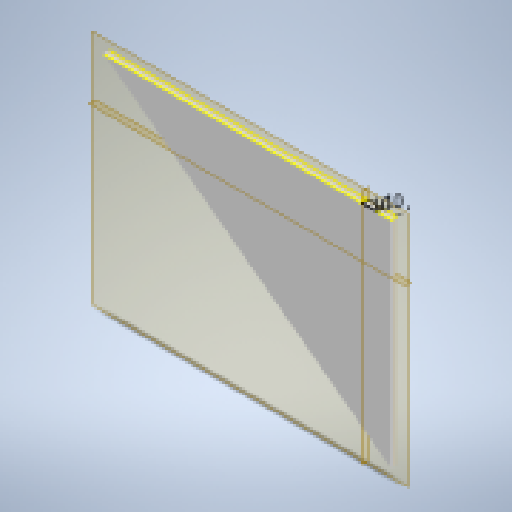
# Autodesk Inventor part: Ребро жёсткости для крепления хвоста
Saved by Autodesk Inventor 2023.2 (Build 272271030, 271C)
## iProperties
Created: 2024-03-15
Part Number: Ребро жёсткости для крепления хвоста
Material: Типовые
Document SubType Name: Modeling
Designer: I9232
Density: 1 g/cm^3
Appearance: По умолчанию
Author: I9232
Autodesk Inventor part; units mm, degrees
sketch "Эскиз1" plane through (0, 0, 0) normal (0, 0, 1) x (1, 0, 0)
  line L0 (-180, 35) -> (20, 35)
  line L1 (20, 35) -> (20, -115)
  line L2 (20, -115) -> (-180, 35)
  dimension "d4" = 150
  dimension "d5" = 200
  constraints: 6 end point, 1 perpendicular
  measures "d4" distance of L0.end L1.end
  measures "d5" distance of L0.start L0.end
extrude "Выдавливание1" add sketch "Эскиз1" along normal mid plane 4
sketch "Эскиз2" plane through (-180, 35, 2) normal (0, 1, 0) x (1, 0, 0)
  line L0 (200, 0) -> (0, 0) projected
  line L1 (0, 4) -> (200, 4) projected
  line L2 (190, 0) -> (180, 0)
  line L3 (180, 0) -> (180, 4)
  line L4 (180, 4) -> (190, 4)
  line L5 (190, 4) -> (190, 0)
  line L6 (200, 4) -> (200, 0) projected
  line L7 (170, 0) -> (160, 0)
  line L8 (160, 0) -> (160, 4)
  line L9 (160, 4) -> (170, 4)
  line L10 (170, 4) -> (170, 0)
  line L11 (-310, 0) -> (-320, 0)
  line L12 (-320, 0) -> (-320, 4)
  line L13 (-320, 4) -> (-310, 4)
  line L14 (-310, 4) -> (-310, 0)
  line L15 (-330, 0) -> (-340, 0)
  line L16 (-340, 0) -> (-340, 4)
  line L17 (-340, 4) -> (-330, 4)
  line L18 (-330, 4) -> (-330, 0)
  line L19 (110, 0) -> (110, 4)
  line L20 (120, 0) -> (110, 0)
  line L21 (110, 4) -> (120, 4)
  line L22 (120, 4) -> (120, 0)
  line L23 (130, 0) -> (130, 4)
  line L24 (130, 4) -> (140, 4)
  line L25 (140, 4) -> (140, 0)
  line L26 (140, 0) -> (130, 0)
  line L27 (60, 0) -> (60, 4)
  line L28 (70, 0) -> (60, 0)
  line L29 (60, 4) -> (70, 4)
  line L30 (70, 4) -> (70, 0)
  line L31 (80, 0) -> (80, 4)
  line L32 (80, 4) -> (90, 4)
  line L33 (90, 4) -> (90, 0)
  line L34 (90, 0) -> (80, 0)
  line L35 (10, 0) -> (10, 4)
  line L36 (20, 0) -> (10, 0)
  line L37 (10, 4) -> (20, 4)
  line L38 (20, 4) -> (20, 0)
  line L39 (30, 0) -> (30, 4)
  line L40 (30, 4) -> (40, 4)
  line L41 (40, 4) -> (40, 0)
  line L42 (40, 0) -> (30, 0)
  point P0 (180, 2)
  point P1 (180, 2)
  point P2 (170, 2)
  point P3 (-320, 2)
  point P4 (-330, 2)
  point P5 (120, 2)
  point P6 (130, 2)
  point P7 (70, 2)
  point P8 (80, 2)
  point P9 (20, 2)
  point P10 (30, 2)
  dimension "d6" = 10
  dimension "d7" = 10
  dimension "d8" = 10
  dimension "d9" = 10
  dimension "d12" = 500
  dimension "d19" = 50
  constraints: 80 end point, 4 horizontal, 4 parallel, 4 point on line, 2 midpoint, 2 perpendicular, 72 other
  measures "d6" distance of L4.end L3.end
  measures "d7" distance between parallel lines of L5 L6
  measures "d8" distance of L9.end L8.end
  measures "d9" distance of point (180, 2) point (170, 2)
  measures "d12" distance of L2.start L11.start
  measures "d19" distance of L2.start L25.end
extrude "Выдавливание2" add sketch "Эскиз2" along normal blind 3 contours L0 L3 L1 L5 | L0 L8 L1 L10 | L0 L23 L1 L25 | L0 L19 L1 L22 | L0 L31 L1 L33 | L0 L27 L1 L30 | L0 L39 L1 L41 | L0 L35 L1 L38
sketch "Эскиз3" plane through (20, -115, 2) normal (1, 0, 0) x (0, 0, -1)
  line L0 (0, 0) -> (0, 150) projected
  line L1 (4, 0) -> (4, 150) projected
  line L2 (0, 11.5) -> (4, 11.5)
  line L3 (4, 11.5) -> (4, 21.5)
  line L4 (4, 21.5) -> (0, 21.5)
  line L5 (0, 21.5) -> (0, 11.5)
  line L6 (0, 0) -> (4, 0) projected
  line L7 (0, 31.5) -> (4, 31.5)
  line L8 (4, 31.5) -> (4, 41.5)
  line L9 (4, 41.5) -> (0, 41.5)
  line L10 (0, 41.5) -> (0, 31.5)
  line L11 (0, 61.5) -> (4, 61.5)
  line L12 (4, 61.5) -> (4, 71.5)
  line L13 (4, 71.5) -> (0, 71.5)
  line L14 (0, 71.5) -> (0, 61.5)
  line L15 (0, 81.5) -> (4, 81.5)
  line L16 (4, 81.5) -> (4, 91.5)
  line L17 (4, 91.5) -> (0, 91.5)
  line L18 (0, 91.5) -> (0, 81.5)
  line L19 (0, 111.5) -> (4, 111.5)
  line L20 (4, 111.5) -> (4, 121.5)
  line L21 (4, 121.5) -> (0, 121.5)
  line L22 (0, 121.5) -> (0, 111.5)
  line L23 (0, 131.5) -> (4, 131.5)
  line L24 (4, 131.5) -> (4, 141.5)
  line L25 (4, 141.5) -> (0, 141.5)
  line L26 (0, 141.5) -> (0, 131.5)
  point P0 (2, 115)
  point P1 (0, 141.5)
  point P2 (0, 91.5)
  point P3 (0, 121.5)
  point P4 (0, 71.5)
  point P5 (0, 61.5)
  point P6 (4, 61.5)
  point P7 (0, 41.5)
  point P8 (4, 31.5)
  point P9 (0, 21.5)
  point P10 (4, 11.5)
  dimension "d26" = 11.5
  dimension "d27" = 10
  dimension "d28" = 10
  dimension "d29" = 10
  dimension "d32" = 50
  constraints: 48 end point, 4 parallel, 4 point on line, 2 horizontal, 2 perpendicular, 1 vertical, 32 other
  measures "d26" distance between parallel lines of L2 L6
  measures "d27" distance of L3.end L2.end
  measures "d28" distance of L9.end L7.start
  measures "d29" distance between parallel lines of L7 L4
  measures "d32" distance of L2.start L11.start
extrude "Выдавливание3" add sketch "Эскиз3" along normal blind 4 contours L0 L4 L1 L2 | L0 L9 L1 L7 | L0 L13 L1 L11 | L0 L17 L1 L15 | L0 L21 L1 L19 | L0 L25 L1 L23
sketch "Эскиз4" plane through (0, 0, 2) normal (0, 0, 1) x (1, 0, 0)
  line L0 (5.1, -89.95) -> (5.1, -87.05)
  line L1 (20, -87.05) -> (20, -89.95)
  line L2 (20, -93.5) -> (20, -83.5) projected
  line L3 (5.1, -88.5) -> (20, -88.5) construction
  line L4 (20, -83.5) -> (20, -93.5) projected
  line L5 (10.1, -91.3) -> (11.9, -91.3)
  line L6 (11.9, -85.7) -> (10.1, -85.7)
  line L7 (20, -89.95) -> (11.9, -89.95)
  line L8 (10.1, -89.95) -> (5.1, -89.95)
  line L9 (10.1, -85.7) -> (10.1, -87.05)
  line L10 (10.1, -89.95) -> (10.1, -91.3)
  line L11 (11.9, -91.3) -> (11.9, -89.95)
  line L12 (11.9, -87.05) -> (11.9, -85.7)
  line L13 (5.1, -87.05) -> (10.1, -87.05)
  line L14 (11.9, -87.05) -> (20, -87.05)
  line L15 (10.1, -39.95) -> (10.1, -41.3)
  line L16 (10.1, -35.7) -> (10.1, -37.05)
  line L17 (10.1, -41.3) -> (11.9, -41.3)
  line L18 (11.9, -41.3) -> (11.9, -39.95)
  line L19 (11.9, -35.7) -> (10.1, -35.7)
  line L20 (11.9, -37.05) -> (11.9, -35.7)
  line L21 (5.1, -38.5) -> (20, -38.5) construction
  line L22 (20, -39.95) -> (11.9, -39.95)
  line L23 (11.9, -37.05) -> (20, -37.05)
  line L24 (20, -37.05) -> (20, -39.95)
  line L25 (5.1, -37.05) -> (10.1, -37.05)
  line L26 (5.1, -39.95) -> (5.1, -37.05)
  line L27 (10.1, -39.95) -> (5.1, -39.95)
  line L28 (10.1, 10.05) -> (10.1, 8.7)
  line L29 (10.1, 14.3) -> (10.1, 12.95)
  line L30 (10.1, 8.7) -> (11.9, 8.7)
  line L31 (11.9, 8.7) -> (11.9, 10.05)
  line L32 (11.9, 14.3) -> (10.1, 14.3)
  line L33 (11.9, 12.95) -> (11.9, 14.3)
  line L34 (5.1, 11.5) -> (20, 11.5) construction
  line L35 (20, 10.05) -> (11.9, 10.05)
  line L36 (11.9, 12.95) -> (20, 12.95)
  line L37 (20, 12.95) -> (20, 10.05)
  line L38 (5.1, 12.95) -> (10.1, 12.95)
  line L39 (5.1, 10.05) -> (5.1, 12.95)
  line L40 (10.1, 10.05) -> (5.1, 10.05)
  line L41 (-6.454, 35) -> (-3.546, 35)
  line L42 (-3.546, 20.1) -> (-6.446, 20.1)
  line L43 (-4.996, 20.1) -> (-5, 35) construction
  line L44 (0, 35) -> (-10, 35) projected
  line L45 (-2.196, 25.1) -> (-2.196, 26.9)
  line L46 (-7.796, 26.9) -> (-7.796, 25.1)
  line L47 (-6.446, 20.1) -> (-6.446, 25.1)
  line L48 (-6.454, 26.9) -> (-6.454, 35)
  line L49 (-7.796, 25.1) -> (-6.446, 25.1)
  line L50 (-3.546, 25.1) -> (-2.196, 25.1)
  line L51 (-2.196, 26.9) -> (-3.546, 26.9)
  line L52 (-6.454, 26.9) -> (-7.796, 26.9)
  line L53 (-3.546, 35) -> (-3.546, 26.9)
  line L54 (-3.546, 25.1) -> (-3.546, 20.1)
  line L55 (-53.546, 25.1) -> (-52.196, 25.1)
  line L56 (-57.796, 26.9) -> (-57.796, 25.1)
  line L57 (-56.454, 26.9) -> (-57.796, 26.9)
  line L58 (-52.196, 25.1) -> (-52.196, 26.9)
  line L59 (-52.196, 26.9) -> (-53.546, 26.9)
  line L60 (-54.996, 20.1) -> (-55, 35) construction
  line L61 (-53.546, 35) -> (-53.546, 26.9)
  line L62 (-56.454, 26.9) -> (-56.454, 35)
  line L63 (-56.454, 35) -> (-53.546, 35)
  line L64 (-53.546, 20.1) -> (-56.446, 20.1)
  line L65 (-53.546, 25.1) -> (-53.546, 20.1)
  line L66 (-56.446, 20.1) -> (-56.446, 25.1)
  line L67 (-57.796, 25.1) -> (-56.446, 25.1)
  line L68 (-103.546, 25.1) -> (-102.196, 25.1)
  line L69 (-107.796, 26.9) -> (-107.796, 25.1)
  line L70 (-106.454, 26.9) -> (-107.796, 26.9)
  line L71 (-102.196, 25.1) -> (-102.196, 26.9)
  line L72 (-102.196, 26.9) -> (-103.546, 26.9)
  line L73 (-104.996, 20.1) -> (-105, 35) construction
  line L74 (-103.546, 35) -> (-103.546, 26.9)
  line L75 (-106.454, 26.9) -> (-106.454, 35)
  line L76 (-106.454, 35) -> (-103.546, 35)
  line L77 (-103.546, 20.1) -> (-106.446, 20.1)
  line L78 (-103.546, 25.1) -> (-103.546, 20.1)
  line L79 (-106.446, 20.1) -> (-106.446, 25.1)
  line L80 (-107.796, 25.1) -> (-106.446, 25.1)
  line L81 (-153.546, 25.1) -> (-152.196, 25.1)
  line L82 (-157.796, 26.9) -> (-157.796, 25.1)
  line L83 (-156.454, 26.9) -> (-157.796, 26.9)
  line L84 (-152.196, 25.1) -> (-152.196, 26.9)
  line L85 (-152.196, 26.9) -> (-153.546, 26.9)
  line L86 (-154.996, 20.1) -> (-155, 35) construction
  line L87 (-153.546, 35) -> (-153.546, 26.9)
  line L88 (-156.454, 26.9) -> (-156.454, 35)
  line L89 (-156.454, 35) -> (-153.546, 35)
  line L90 (-153.546, 20.1) -> (-156.446, 20.1)
  line L91 (-153.546, 25.1) -> (-153.546, 20.1)
  line L92 (-156.446, 20.1) -> (-156.446, 25.1)
  line L93 (-157.796, 25.1) -> (-156.446, 25.1)
  point P0 (0, 0)
  point P1 (11.9, -86.375)
  point P2 (11.9, -90.625)
  point P3 (11.9, -40.625)
  point P4 (11.9, -36.375)
  point P5 (11.9, 9.375)
  point P6 (11.9, 13.625)
  point P7 (-7.125, 26.9)
  point P8 (-57.125, 26.9)
  point P9 (-107.125, 26.9)
  point P10 (-157.125, 26.9)
  dimension "d39" = 2.9
  dimension "d40" = 5.6
  dimension "d41" = 1.8
  dimension "d43" = 5
  dimension "d44" = 8.1
  dimension "d45" = 8.1
  dimension "d46" = 1.35
  dimension "d49" = 50
  dimension "d54" = 2.9
  dimension "d55" = 1.8
  dimension "d56" = 5.6
  dimension "d57" = 1.35
  dimension "d58" = 5
  dimension "d59" = 8.1
  dimension "d62" = 50
  constraints: 182 end point, 24 parallel, 9 midpoint, 9 perpendicular, 7 horizontal, 1 vertical, 142 other
  measures "d39" distance of L0.start L0.end
  measures "d40" distance between parallel lines of L6 L5
  measures "d41" distance of L6.start L6.end
  measures "d43" distance of L9.end L0.end
  measures "d44" distance from line of L1 point (11.9, -86.375)
  measures "d45" distance from line of L2 point (11.9, -90.625)
  measures "d46" distance of L8.start L5.start
  measures "d49" distance of L5.start L15.end
  measures "d54" distance of L42.start L42.end
  measures "d55" distance of L46.start L46.end
  measures "d56" distance of L45.end L46.start
  measures "d57" distance of L46.end L47.end
  measures "d58" distance of L42.end L47.end
  measures "d59" distance from line of L44 point (-7.125, 26.9)
  measures "d62" distance of L45.start L55.end
extrude "Выдавливание4" cut sketch "Эскиз4" against normal up to surface (4 mm away)
